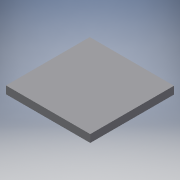
# Autodesk Inventor part: motor holder
Saved by Autodesk Inventor 2016 (Build 200138000, 138)
## iProperties
Created: 2017-01-30
Part Number: motor holder
Material: Generic
Document SubType Name: Modeling
Designer: student1
Density: 1 g/cm^3
Appearance: Default
Author: student1
Autodesk Inventor part; units mm, degrees
ref_plane "YZ Plane" through (0, 0, 0) normal (1, 0, 0) x (0, 1, 0)
ref_plane "XZ Plane" through (0, 0, 0) normal (0, 1, 0) x (-1, 0, 0)
ref_plane "XY Plane" through (0, 0, 0) normal (0, 0, 1) x (1, 0, 0)
sketch "Sketch1" plane through (0, 0, 0) normal (0, 1, 0) x (-1, 0, 0)
  line L0 (22.3834, 76.1397) -> (-79.2166, 76.1397)
  line L1 (-79.2166, 76.1397) -> (-79.2166, -25.4603)
  line L2 (-79.2166, -25.4603) -> (22.3834, -25.4603)
  line L3 (22.3834, -25.4603) -> (22.3834, 76.1397)
  point P0 (0, 0)
  dimension "d0" = 101.6
  dimension "d1" = 101.6
  constraints: 8 end point, 2 parallel, 1 horizontal, 1 perpendicular
  measures "d0" distance of L2.end L0.start
  measures "d1" distance of L1.end L2.end
extrude "Extrusion1" add sketch "Sketch1" along normal blind 2.54
sketch "Sketch2" plane through (0, 0, 0) normal (0, -1, 0) x (1, 0, 0)
  line L0 (-22.3834, 76.1397) -> (79.2166, 76.1397) projected
  line L1 (79.2166, -25.4603) -> (-22.3834, -25.4603) projected
  line L2 (51.0699, 76.1397) -> (-22.3834, 76.1397)
  line L3 (-22.3834, 76.1397) -> (-22.3834, -25.4603)
  line L4 (-22.3834, -25.4603) -> (51.0699, -25.4603)
  line L5 (51.0699, -25.4603) -> (51.0699, 76.1397)
  point P0 (0, 0)
  constraints: 8 end point, 2 parallel, 1 horizontal, 1 perpendicular, 1 point on line
extrude "Extrusion2" cut sketch "Sketch2" against normal blind 25.4
sketch "Sketch3" plane through (0, 0, 0) normal (0, -1, 0) x (1, 0, 0)
  line L0 (79.2166, 76.1397) -> (79.2166, -25.4603) projected
  line L1 (51.0699, -25.4603) -> (51.0699, 76.1397) projected
  line L2 (79.2166, 48.1612) -> (51.0699, 48.1612)
  line L3 (51.0699, 48.1612) -> (51.0699, -25.4603)
  line L4 (51.0699, -25.4603) -> (79.2166, -25.4603)
  line L5 (79.2166, -25.4603) -> (79.2166, 48.1612)
  point P0 (0, 0)
  constraints: 8 end point, 2 parallel, 1 horizontal, 1 perpendicular, 1 point on line
extrude "Extrusion3" cut sketch "Sketch3" against normal blind 25.4
equation "\"d1\" = d0"
body "Solid1"
